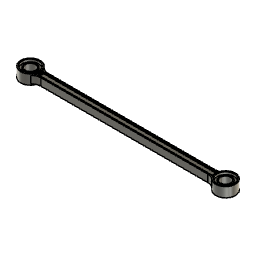
Leading Wheel Link (Autodesk Fusion 360 design; units mm, degrees)
Autodesk Fusion 360 part; units mm, degrees
sketch "Sketch1" plane through (0, 0, 0) normal (0, 0, 1) x (1, 0, 0) in component "Component"
  circle A0 centre (0, 0) radius 1.05
  circle A1 centre (0, 0) radius 1.25
  circle A2 centre (0, 0) radius 2
  circle A3 centre (0, 0) radius 1.75
  circle A4 centre (40, 0) radius 1.05
  circle A5 centre (40, 0) radius 1.25
  circle A6 centre (40, 0) radius 2
  circle A7 centre (40, 0) radius 1.75
  arc A8 (37.6548, 0.375) -> (37.6548, -0.375) centre (40, 0) ccw
  line L0 (1.5811, -0.75) -> (38.146, -0.75)
  line L1 (2.3452, -0.375) -> (37.6548, -0.375)
  line L2 (2.3452, 0.375) -> (37.6548, 0.375)
  line L3 (38.146, 0.75) -> (1.854, 0.75)
  arc A9 (2.3452, -0.375) -> (2.3452, 0.375) centre (0, 0) ccw
  line L4 (2.0976, -0.575) -> (37.9024, -0.575)
  arc A10 (37.9024, 0.575) -> (37.9024, -0.575) centre (40, 0) ccw
  line L5 (2.0976, 0.575) -> (37.9024, 0.575)
  arc A11 (2.0976, -0.575) -> (2.0976, 0.575) centre (0, 0) ccw
  point P0 (40, 0)
  dimension "d1" = 2.1
  dimension "d2" = 2.5
  dimension "d3" = 4
  dimension "d4" = 3.5
  dimension "d7" = 40
  dimension "d8" = 0
  dimension "d16" = -0.2
  constraint coincident A0.centre A1.centre
  constraint concentric A0 A2
  constraint concentric A0 A3
  constraint coincident A6 L3.start
  constraint coincident A6 L0.end
  constraint concentric A6 A8
  constraint coincident A3 L0.start
  constraint coincident A2 L3.end
  constraint concentric A2 A9
  measures "d1" diameter of A0
  measures "d2" diameter of A1
  measures "d3" diameter of A2
  measures "d4" diameter of A3
extrude "Extrude1" add sketch "Sketch1" along normal blind 2 contours A2 | A6 makes body 1 at (40.5417, 1.9252, 1.3333) makes body 2 at (1.9901, 0.1991, 1.3333) in component "Component"
extrude "Extrude2" add sketch "Sketch1" along normal blind 1.75 separate body contours A1 | A5 makes body 3 at (1.2438, -0.1245, 1.1667) makes body 4 at (41.2438, -0.1245, 1.1667) in component "Component"
extrude "Extrude3" cut sketch "Sketch1" along normal blind 0.25 contours A1 | A5 bodies 3 4 in component "Component"
extrude "Extrude4" add sketch "Sketch1" along normal blind 1.5 contours A3 | A7 bodies 1 2 3 4 in component "Component"
extrude "Extrude5" cut sketch "Sketch1" along normal blind 0.5 contours A3 | A7 bodies 1 2 in component "Component"
extrude "Extrude6" add sketch "Sketch1" along normal blind 1.75 contours A2 A6 L0 L3 bodies 1 2 in component "Component"
extrude "Extrude7" cut sketch "Sketch1" along normal blind 0.25 contours A2 A6 L0 L3 bodies 1 in component "Component"
extrude "Extrude8" add sketch "Sketch1" along normal blind 1.625 separate body contours A8 L1 L2 A9 makes body 5 in component "Component"
extrude "Extrude9" cut sketch "Sketch1" along normal blind 0.375 contours A8 L1 L2 A9 bodies 5 in component "Component"
extrude "Extrude10" add sketch "Sketch1" along normal blind 1.5 contours L4 A10 L5 A11 bodies 1 5 in component "Component"
extrude "Extrude11" cut sketch "Sketch1" along normal blind 0.5 contours L4 A10 L5 A11 bodies 1 in component "Component"
fillet "Fillet1" radius 2 4 edges at (1.854, -0.75, 1) (38.146, -0.75, 1) (1.854, 0.75, 1) (38.146, 0.75, 1) on bodies 1 in component "Component"
component "Component" placed x (1, 0, 0) y (0, 1, 0) z (0, 0, 1) at (0, 0, 0)
